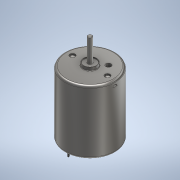
# Autodesk Inventor part: motor
Saved by Autodesk Inventor 2022 (Build 260153000, 153)
## iProperties
Created: 2018-03-11
Part Number: motor
Material: Stainless Steel
Document SubType Name: Modeling
Designer: basil
Density: 8 g/cm^3
Appearance: Semi-Polished
Author: basil
Autodesk Inventor part; units mm, degrees
ref_plane "XZ Plane" through (0, 0, 0) normal (0, 1, 0) x (-1, 0, 0)
ref_plane "XY Plane" through (0, 0, 0) normal (0, 0, 1) x (1, 0, 0)
sketch "Sketch1" plane through (0, 0, 0) normal (0, 0, 1) x (1, 0, 0)
  circle A0 centre (0, 0) radius 12.2
  dimension "d0" = 24.4
  constraints: 1 centre point, 1 coincident
  measures "d0" diameter of A0
extrude "Extrusion1" add sketch "Sketch1" along normal blind 30.8
fillet "Fillet1" radius 1 1 edges at (-12.2, 0, 30.8)
sketch "Sketch4" plane through (0, 0, 30.8) normal (0, 0, 1) x (1, 0, 0)
  circle A0 centre (0, 0) radius 3.2
  circle A1 centre (0, 0) radius 3
  dimension "d10" = 6.4
  dimension "d11" = 6
  constraints: 2 centre point, 2 coincident
  measures "d10" diameter of A0
  measures "d11" diameter of A1
extrude "Extrusion4" add sketch "Sketch4" along normal blind 1.5
fillet "Fillet2" radius 0.25 1 edges at (-3.2, 0, 30.8)
sketch "Sketch6" plane through (0, 0, 30.8) normal (0, 0, 1) x (1, 0, 0)
  circle A0 centre (0, 0) radius 2.9
  circle A1 centre (0, 0) radius 1.1
  dimension "d18" = 5.8
  dimension "d19" = 2.2
  constraints: 2 centre point, 2 coincident
  measures "d18" diameter of A0
  measures "d19" diameter of A1
extrude "Extrusion6" add sketch "Sketch6" along normal blind 1.2
sketch "Sketch7" plane through (0, 0, 30.8) normal (0, 0, 1) x (1, 0, 0)
  circle A0 centre (0, 0) radius 1
  dimension "d22" = 2
  constraints: 1 centre point, 1 coincident
  measures "d22" diameter of A0
extrude "Extrusion7" add sketch "Sketch7" along normal blind 12.5
sketch "Sketch8" plane through (0, 0, 30.8) normal (0, 0, 1) x (1, 0, 0)
  line L0 (0, 0) -> (8.5, 0)
  dimension "d26" = 8.5
  constraints: 2 end point, 1 horizontal
  measures "d26" distance of L0.start L0.end
hole "Hole1" at (8.5, 0, 30.8) direction (0, 0, -1) diameter 2.459 depth 0.8 tip angle 118 thread size "M3x0.5" class "6H" standard "ANSI Metric M Profile"
pattern_circular "Circular Pattern1" count 2 over 360 about axis through (0, 0, 43.3) along (0, 0, 1) of "Hole1"
sketch "Sketch9" plane through (0, 0, 30.8) normal (0, 0, 1) x (1, 0, 0)
  circle A0 centre (4.3293, 4.6166) radius 1.25
  point P0 (0, 0)
  dimension "d37" = 2.5
  constraints: 1 centre point
  measures "d37" diameter of A0
extrude "Extrusion8" cut sketch "Sketch9" against normal blind 2
ref_plane "Work Plane1" through (12.25, 0, 0) normal (1, 0, 0) x (0, 1, 0)
sketch "Sketch10" plane through (12.25, 0, 0) normal (1, 0, 0) x (0, 1, 0)
  arc A0 (1, 27.9762) -> (-1, 27.9762) centre (0, 27.9762) ccw
  line L0 (0, 27.9762) -> (1, 27.9762)
  line L1 (0, 27.9762) -> (-1, 27.9762)
  point P0 (0, 0)
  dimension "d41" = 2
  constraints: 4 end point, 2 point on circle, 1 centre point, 1 horizontal
  measures "d41" diameter of A0
extrude "Extrusion9" cut sketch "Sketch10" against normal blind 1
pattern_circular "Circular Pattern2" count 2 over 360 about axis through (0, 0, 43.3) along (0, 0, 1) of "Extrusion9"
sketch "Sketch11" plane through (0, 0, 0) normal (0, 0, -1) x (-1, 0, 0)
  circle A0 centre (0, 0) radius 3.2 projected
  circle A1 centre (0, 0) radius 3.2
  circle A2 centre (0, 0) radius 3.1
  dimension "d47" = 6.4
  dimension "d48" = 6.2
  constraints: 2 centre point, 2 coincident
  measures "d47" diameter of A1
  measures "d48" diameter of A2
extrude "Extrusion10" add sketch "Sketch11" along normal blind 1
sketch "Sketch12" plane through (0, 0, 0) normal (0, 0, -1) x (-1, 0, 0)
  circle A0 centre (0, 0) radius 1
  dimension "d51" = 2
  constraints: 1 centre point, 1 coincident
  measures "d51" diameter of A0
extrude "Extrusion11" add sketch "Sketch12" along normal blind 0.5
sketch "Sketch13" plane through (0, 0, -0.5) normal (0, 0, -1) x (-1, 0, 0)
  circle A0 centre (0, 0) radius 2.75
  dimension "d54" = 5.5
  constraints: 1 centre point, 1 coincident
  measures "d54" diameter of A0
extrude "Extrusion12" add sketch "Sketch13" along normal blind 1
sketch "Sketch14" plane through (0, 0, -1.5) normal (0, 0, -1) x (-1, 0, 0)
  circle A0 centre (0, 0) radius 2
  circle A1 centre (0, 0) radius 1.9
  dimension "d57" = 4
  dimension "d58" = 3.8
  constraints: 2 centre point, 2 coincident
  measures "d57" diameter of A0
  measures "d58" diameter of A1
extrude "Extrusion13" cut sketch "Sketch14" against normal blind 0.5
sketch "Sketch15" plane through (0, 0, -1.5) normal (0, 0, -1) x (-1, 0, 0)
  circle A0 centre (0, 0) radius 2 projected
  circle A1 centre (0, 0) radius 0.5
  dimension "d61" = 1
  constraints: 1 centre point, 1 coincident
  measures "d61" diameter of A1
extrude "Extrusion14" cut sketch "Sketch15" against normal blind 1 contours A1
sketch "Sketch16" plane through (0, 0, 0) normal (0, 0, -1) x (-1, 0, 0)
  line L0 (0, 4.25) -> (0, 4.25)
  line L1 (0, 4.25) -> (0, 4.25)
  circle A0 centre (0, 0) radius 2 projected
  arc A1 (-1.2481, -3.5362) -> (1.2481, -3.5362) centre (0, 0) ccw
  arc A2 (1.2481, 3.5362) -> (-1.2481, 3.5362) centre (0, 0) ccw
  arc A3 (-1.4145, -4.0077) -> (1.4145, -4.0077) centre (0, 0) ccw
  arc A4 (1.4145, 4.0077) -> (-1.4145, 4.0077) centre (0, 0) ccw
  line L2 (0, 0) -> (-0.6656, -1.886)
  line L3 (-1.2481, -3.5362) -> (-1.4145, -4.0077)
  line L4 (0, 0) -> (0.6656, -1.886)
  line L5 (1.2481, -3.5362) -> (1.4145, -4.0077)
  line L6 (1.4145, 4.0077) -> (1.2481, 3.5362)
  line L7 (0.6656, 1.886) -> (0, 0)
  line L8 (-1.4145, 4.0077) -> (-1.2481, 3.5362)
  line L9 (-0.6656, 1.886) -> (0, 0)
  dimension "d66" = 0
  dimension "d67" = 0
  constraints: 20 end point, 13 point on circle, 4 centre point, 2 coincident, 2 horizontal, 2 tangent
  measures "d66" distance of L0.start L0.end
  measures "d67" distance of L0.start L1.end
extrude "Extrusion15" cut sketch "Sketch16" against normal blind 2 contours A1 L5 A3 L3 | A2 L8 A4 L6
sketch "Sketch17" plane through (0, 0, 0) normal (0, 0, -1) x (-1, 0, 0)
  circle A0 centre (0, 0) radius 0.5 projected
  circle A1 centre (0, 0) radius 11.2 projected
  line L0 (0, 11) -> (1.5, 11)
  line L1 (0, 10) -> (1.5, 10)
  line L2 (0, 11) -> (-1.5, 11)
  line L3 (0, 10) -> (-1.5, 10)
  arc A2 (1.5, 10) -> (1.5, 11) centre (1.3547, 10.5) ccw
  arc A3 (-1.5, 11) -> (-1.5, 10) centre (-1.3891, 10.5) ccw
  circle A4 centre (2.6692, 10.1025) radius 0.5
  circle A5 centre (-2.6604, 10.1025) radius 0.5
  dimension "d70" = 10
  dimension "d71" = 1
  dimension "d74" = 1.5
  dimension "d77" = 1.5
  dimension "d78" = 1
  dimension "d79" = 1
  constraints: 8 end point, 4 centre point, 4 horizontal, 4 point on circle
  measures "d70" distance of A0.centre L1.start
  measures "d71" distance of L1.start L0.start
  measures "d74" distance of L0.start L0.end
  measures "d77" distance of L1.start L3.end
  measures "d78" diameter of A4
  measures "d79" diameter of A5
extrude "Extrusion16" add sketch "Sketch17" along normal blind 0.25 contours L0 A2 L1 L3 A3 L2 | A4 | A5
pattern_circular "Circular Pattern3" count 2 over 360 about axis through (0, 0, 43.3) along (0, 0, 1) of "Extrusion16"
fillet "Fillet3" radius 1 1 edges at (-12.2, 0, 0)
sketch "Sketch18" plane through (0, 0, 0) normal (0, 0, -1) x (-1, 0, 0)
  circle A0 centre (5.4492, 2.1432) radius 0.5
  point P0 (0, 0)
  dimension "d86" = 1
  constraints: 1 centre point
  measures "d86" diameter of A0
extrude "Extrusion17" cut sketch "Sketch18" against normal blind 1
pattern_circular "Circular Pattern4" count 2 over 360 about axis through (0, 0, 43.3) along (0, 0, 1) of "Extrusion17"
sketch "Sketch19" plane through (0, 0, -0.25) normal (0, 0, -1) x (-1, 0, 0)
  line L0 (0, 10.8419) -> (0.2, 10.8419)
  line L1 (0.2, 10.8419) -> (0.2, 10.1641)
  line L2 (0.2, 10.1641) -> (0, 10.1641)
  line L3 (0, 10.1641) -> (0, 10.8419)
  point P0 (0, 0)
  dimension "d92" = 0.2
  constraints: 8 end point, 2 parallel, 1 horizontal, 1 perpendicular
  measures "d92" distance of L1.end L2.end
extrude "Extrusion18" add sketch "Sketch19" along normal blind 2
sketch "Sketch20" plane through (0, 10.1641, -0.25) normal (1, 0, 0) x (0, 0, -1)
  circle A0 centre (1.6987, 0.3388) radius 0.15
  line L0 (0, -0.1641) -> (0, 0.8359) projected
  line L1 (0, 0.4888) -> (1.2018, 0.4888)
  line L2 (1.2018, 0.4888) -> (1.2018, 0.1888)
  line L3 (1.2018, 0.1888) -> (0, 0.1888)
  line L4 (0, 0.1888) -> (0, 0.4888)
  point P0 (-0.25, -10.1641)
  dimension "d95" = 0.3
  constraints: 8 end point, 2 parallel, 1 centre point, 1 horizontal, 1 perpendicular, 1 point on line
  measures "d95" diameter of A0
extrude "Extrusion19" cut sketch "Sketch20" along normal mid plane 4
fillet "Fillet4" radius 0.25 2 edges at (-0.1, 10.8419, -2.25) (-0.1, 10.1641, -2.25)
pattern_circular "Circular Pattern5" count 2 over 360 about axis through (0, 0, 43.3) along (0, 0, 1) of "Extrusion18", "Extrusion19"
fillet "Fillet5" radius 0.25 2 edges at (0.1, -10.1641, -2.25) (0.1, -10.8419, -2.25)
fillet "Fillet6" radius 0.25 1 edges at (2.75, 0, -1.5)
fillet "Fillet7" radius 0.25 1 edges at (-1, 0, 43.3)
body "Solid1"
